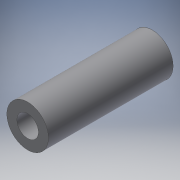
# Autodesk Inventor part: XMotorStandoff
Saved by Autodesk Inventor 2019 (Build 230136000, 136)
## iProperties
Created: 2018-10-21
Part Number: XMotorStandoff
Material: Generic
Document SubType Name: Modeling
Designer: LillaHunden
Density: 1 g/cm^3
Appearance: Default
Author: LillaHunden
Autodesk Inventor part; units mm, degrees
ref_plane "YZ Plane" through (0, 0, 0) normal (1, 0, 0) x (0, 1, 0)
ref_plane "XZ Plane" through (0, 0, 0) normal (0, 1, 0) x (-1, 0, 0)
ref_plane "XY Plane" through (0, 0, 0) normal (0, 0, 1) x (1, 0, 0)
sketch "Sketch1" plane through (0, 0, 0) normal (0, 0, 1) x (1, 0, 0)
  circle A0 centre (17.9351, 49.0714) radius 2.6 construction
  circle A1 centre (17.9351, 49.0714) radius 5
  circle A2 centre (17.9351, 49.0714) radius 2.6
  point P0 (0, 0)
  dimension "d0" = 10
  constraints: 2 centre point, 2 coincident, 1 concentric
  measures "d0" diameter of A1
ref_plane "Work Plane1" through (-33.1349, -1.9986, 30) normal (0, 0, -1) x (0, 1, 0)
extrude "Extrusion1" add sketch "Sketch1" along normal up to surface (30 mm away)
body "Solid1"
